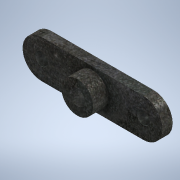
# Autodesk Inventor part: Крышка
Saved by Autodesk Inventor 2020 (Build 240168000, 168)
## iProperties
Created: 2022-04-06
Part Number: Крышка
Material: Сталь
Document SubType Name: Modeling
Designer: User
Density: 7.85 g/cm^3
Appearance: Листовая
Author: User
Autodesk Inventor part; units mm, degrees
ref_plane "YZ Plane" through (0, 0, 0) normal (1, 0, 0) x (0, 1, 0)
ref_plane "XZ Plane" through (0, 0, 0) normal (0, 1, 0) x (-1, 0, 0)
ref_plane "XY Plane" through (0, 0, 0) normal (0, 0, 1) x (1, 0, 0)
sketch "Эскиз1" plane through (0, 0, 0) normal (0, 0, 1) x (1, 0, 0)
  line L0 (-40, 0) -> (40, 0) construction
  line L1 (-40, -15) -> (40, -15)
  line L2 (40, 15) -> (-40, 15)
  arc A0 (-40, 15) -> (-40, -15) centre (-40, 0) ccw
  arc A1 (40, -15) -> (40, 15) centre (40, 0) ccw
  circle A2 centre (0, 0) radius 12.5
  circle A3 centre (-40, 0) radius 5
  circle A4 centre (40, 0) radius 5
  circle A5 centre (0, 0) radius 6
  dimension "d0" = 40
  dimension "d1" = 30
  dimension "d4" = 25
  dimension "d5" = 10
  dimension "d6" = 10
  dimension "d7" = 12
  constraints: 8 end point, 6 centre point, 4 point on circle, 4 tangent, 3 coincident, 1 concentric, 1 horizontal, 1 midpoint, 1 parallel
  measures "d0" distance of point (0, 0) L0.end
  measures "d1" diameter of A1
  measures "d4" diameter of A2
  measures "d5" diameter of A3
  measures "d6" diameter of A4
  measures "d7" diameter of A5
extrude "Выдавливание1" add sketch "Эскиз1" along normal blind 8 contours A0 L2 A1 L1 | A2 | A3 | A4 | A5
extrude "Выдавливание2" cut sketch "Эскиз1" along normal through all contours A3 | A4
extrude "Выдавливание3" cut sketch "Эскиз1" along normal blind 20 contours A5
extrude "Выдавливание4" add sketch "Эскиз1" along normal blind 20 contours A2
